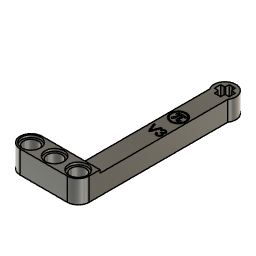
1. Stepper motor holder (L) [V3] (Autodesk Fusion 360 design; units mm, degrees)
Autodesk Fusion 360 part; units mm, degrees
note: some values were not read from the file. Set by a fixed rule: which sketch regions a step uses.
sketch "Base" plane through (0, 0, 0) normal (0, 0, 1) x (1, 0, 0)
  line L0 (3.7, 0) -> (19.7, 0)
  line L1 (19.7, 7.4) -> (3.7, 7.4)
  arc A0 (3.7, 7.4) -> (0, 3.7) centre (3.7, 3.7) ccw
  arc A1 (0, 3.7) -> (3.7, 0) centre (3.7, 3.7) ccw
  arc A2 (19.7, 0) -> (23.4, 3.7) centre (19.7, 3.7) ccw
  circle A3 centre (3.7, 3.7) radius 2.5
  circle A4 centre (3.7, 3.7) radius 3.2
  circle A5 centre (11.7, 3.7) radius 2.5
  circle A6 centre (11.7, 3.7) radius 3.2
  circle A7 centre (19.7, 3.7) radius 2.5
  circle A8 centre (19.7, 3.7) radius 3.2
  line L2 (19.7, 7.4) -> (23.4, 7.4)
  line L3 (23.4, 7.4) -> (23.4, 3.7)
  line L4 (17.85, 52.8) -> (22.85, 52.8)
  line L5 (20.35, 55.3003) -> (20.35, 50.2997)
  line L6 (17.85, 52.8) -> (17.85, 51.75)
  line L7 (19.3, 50.2997) -> (20.35, 50.2997)
  line L8 (20.35, 54.8003) -> (20.35, 0.0575)
  circle A9 centre (20.35, 52.8) radius 3.7125
  line L9 (23.4, 51.75) -> (23.4, 7.4)
  line L10 (17.3, 51.75) -> (17.3, 7.4)
  line L11 (17.85, 51.75) -> (19.05, 51.75)
  line L12 (19.3, 51.5) -> (19.3, 50.2997)
  arc A10 (19.3, 51.5) -> (19.05, 51.75) centre (19.05, 51.5) ccw
  line L13 (22.85, 52.8) -> (22.85, 51.75)
  line L14 (22.85, 51.75) -> (21.65, 51.75)
  arc A11 (21.65, 51.75) -> (21.4, 51.5) centre (21.65, 51.5) ccw
  line L15 (21.4, 51.5) -> (21.4, 50.2997)
  line L16 (21.4, 50.2997) -> (20.35, 50.2997)
  line L17 (17.85, 52.8) -> (17.85, 53.85)
  line L18 (17.85, 53.85) -> (19.05, 53.85)
  arc A12 (19.05, 53.85) -> (19.3, 54.1) centre (19.05, 54.1) ccw
  line L19 (19.3, 54.1) -> (19.3, 55.3003)
  line L20 (19.3, 55.3003) -> (20.35, 55.3003)
  line L21 (21.4, 55.3003) -> (20.35, 55.3003)
  line L22 (21.4, 54.1) -> (21.4, 55.3003)
  arc A13 (21.4, 54.1) -> (21.65, 53.85) centre (21.65, 54.1) ccw
  line L23 (22.85, 53.85) -> (21.65, 53.85)
  line L24 (22.85, 52.8) -> (22.85, 53.85)
  line L25 (17.3, 51.75) -> (17.3, 52.75)
  line L26 (23.4, 51.75) -> (23.4, 52.75)
  arc A14 (20.35, 55.8) -> (17.3, 52.75) centre (20.35, 52.75) ccw
  arc A15 (23.4, 52.75) -> (20.35, 55.8) centre (20.35, 52.75) ccw
  point P0 (23.4, 0)
  point P1 (0, 7.4)
  point P2 (17.3, 54.8)
  point P3 (17.3, 55.8)
  point P4 (23.4, 55.8)
  dimension "d1" = 23.4
  dimension "d2" = 7.4
  dimension "d3" = 3.7
  dimension "d4" = 3.7
  dimension "d6" = 3.7
  dimension "d7" = 5
  dimension "d8" = 6.4
  dimension "d11" = 16
  dimension "d12" = 0
  dimension "d50" = 1.05
  dimension "d51" = 1.05
  dimension "d58" = 0.25
  dimension "d61" = 3.05
  dimension "d62" = 3.05
  constraint horizontal L0
  constraint horizontal L1
  constraint coincident P1 L1
  constraint tangent L1 A0
  constraint coincident origin L0
  constraint tangent L0 A1
  constraint coincident A0.end A1.start
  constraint coincident P0 L0
  constraint tangent L0 A2
  constraint concentric A1 A3
  constraint concentric A0 A4
  constraint horizontal L2
  constraint vertical L3
  constraint midpoint L4 L5
  constraint perpendicular L4 L6
  constraint coincident A2 L8.end
  constraint perpendicular L0 L8
  constraint perpendicular L4 L5
  constraint parallel L5 L8
  constraint midpoint L4 A9.centre
  constraint coincident L1 L10.end
  constraint perpendicular L1 L10
  constraint perpendicular L6 L11
  constraint tangent L11 A10
  constraint tangent L12 A10
  constraint symmetric L4.start L8 L4.end
  constraint symmetric L5.end L8 L7.end
  constraint symmetric L6.end L8 L13.end
  constraint symmetric L7.start L8 L15.end
  constraint symmetric L8 L11.end L14.end
  constraint symmetric L8 L12.start A11.end
  constraint symmetric L8 A10 A11
  constraint symmetric L6.start L4 L17.start
  constraint symmetric L4 L5.end L5.start
  constraint symmetric L4 L6.end L17.end
  constraint symmetric L4 L7.start L19.end
  constraint symmetric L4 L11.end L18.end
  constraint symmetric L4 L12.start A12.end
  constraint symmetric L4 A10 A12
  constraint symmetric L4 L13.start L24.start
  constraint symmetric L4 L13.end L23.start
  constraint symmetric L4 L14.end A13.end
  constraint symmetric L4 A11.end L22.start
  constraint symmetric L4 A11 A13
  constraint symmetric L4 L15.end L21.start
  constraint parallel L10 L25
  constraint parallel L9 L26
  constraint coincident P3 L25
  constraint tangent L25 A14
  constraint coincident P4 L26
  constraint tangent L26 A15
  constraint coincident A14.start A15.end
  measures "d1" distance of origin P0
  measures "d2" distance of origin P1
  measures "d3" radius of A0
  measures "d4" radius of A1
  measures "d6" radius of A2
  measures "d7" diameter of A3
  measures "d8" diameter of A4
  measures "d50" distance of L5.end L7.start
  measures "d51" distance of L4.start L6.end
  measures "d58" radius of A10
  measures "d61" radius of A14
  measures "d62" radius of A15
extrude "Extrude1" add sketch "Base" along normal blind 7.7 contours L0 L1 A0 A1 A2 A8 L2 L8 | A2 A8 L2 L3 L8
extrude "Extrude2" add sketch "Base" along normal blind 6.9 contours A7 A8 L8 | A7 A8 L8 | A4 | A6
extrude "Extrude3" cut sketch "Base" along normal blind 0.8 contours A7 A8 L8 | A7 A8 L8 | A4 | A6
extrude "Extrude4" add sketch "Base" along normal blind 6.7 contours L1 L2 L8 A9 L10 | L2 L8 A9 L9 | A9 L9 L10 L25 L26 A14 A15 | A9 L9 L10 L25 L26 A14 A15
ref_plane "WorkPlane1" through (20.35, 32.5818, 6.7) normal (0, 0, 1) x (1, 0, 0)
sketch "Author" plane through (0, 0, 6.7) normal (0, 0, 1) x (1, 0, 0)
  line L0 (18.8552, 37.6405) -> (18.9613, 37.6326)
  spline S0 degree 3 poles (18.9613, 37.6326) (19.0712, 37.757) (19.1144, 38.1249) (19.7625, 38.0529) knots 0 0 0 0 1 1 1 1
  spline S1 degree 3 poles (19.7625, 38.0529) (19.7389, 36.4766) (19.0477, 36.3103) (19.0909, 35.9869) knots 0 0 0 0 1 1 1 1
  spline S2 degree 3 poles (19.0909, 35.9869) (19.1066, 35.8036) (19.2519, 35.691) (19.409, 35.6845) knots 0 0 0 0 1 1 1 1
  spline S3 degree 3 poles (19.409, 35.6845) (19.9052, 35.7015) (19.883, 36.3705) (20.0374, 38.0568) knots 0 0 0 0 1 1 1 1
  line L1 (20.0374, 38.0568) -> (20.6777, 38.0568)
  spline S4 degree 3 poles (20.6777, 38.0568) (20.6436, 37.4624) (20.5507, 36.868) (20.5402, 36.2854) knots 0 0 0 0 1 1 1 1
  spline S5 degree 3 poles (20.5402, 36.2854) (20.548, 35.8979) (20.7837, 35.691) (21.094, 35.6884) knots 0 0 0 0 1 1 1 1
  spline S6 degree 3 poles (21.094, 35.6884) (21.6046, 35.6714) (21.7656, 36.2671) (21.7656, 36.5211) knots 0 0 0 0 1 1 1 1
  line L2 (21.7656, 36.5211) -> (21.6556, 36.5211)
  spline S7 degree 3 poles (21.6556, 36.5211) (21.6452, 36.3116) (21.5444, 36.161) (21.3297, 36.1519) knots 0 0 0 0 1 1 1 1
  spline S8 degree 3 poles (21.3297, 36.1519) (20.7444, 36.144) (21.0665, 37.1809) (21.0704, 38.0489) knots 0 0 0 0 1 1 1 1
  line L3 (21.0704, 38.0489) -> (21.7656, 38.045)
  line L4 (21.7656, 38.045) -> (21.7617, 38.4888)
  spline S9 degree 3 poles (21.7617, 38.4888) (18.8722, 38.5028) (19.2389, 38.5595) (18.8552, 37.6405) knots 0 0 0 0 1 1 1 1
  arc A0 (17.6646, 37.0896) -> (20.3104, 39.7354) centre (20.3104, 37.0896) cw
  arc A1 (20.3104, 34.4438) -> (17.6646, 37.0896) centre (20.3104, 37.0896) cw
  arc A2 (22.9562, 37.0896) -> (20.3104, 34.4438) centre (20.3104, 37.0896) cw
  arc A3 (20.3104, 39.7354) -> (22.9562, 37.0896) centre (20.3104, 37.0896) cw
  arc A4 (20.3104, 39.3815) -> (20.3694, 39.3807) centre (20.3107, 37.0896) cw
  arc A5 (20.3694, 39.3807) -> (20.4284, 39.3784) centre (20.3103, 37.0896) cw
  arc A6 (20.4284, 39.3784) -> (20.4873, 39.3746) centre (20.3102, 37.0896) cw
  arc A7 (20.4873, 39.3746) -> (20.5461, 39.3693) centre (20.3107, 37.0896) cw
  arc A8 (20.5461, 39.3693) -> (20.6047, 39.3625) centre (20.3104, 37.0896) cw
  arc A9 (20.6047, 39.3625) -> (20.6631, 39.3542) centre (20.3106, 37.0896) cw
  arc A10 (20.6631, 39.3542) -> (20.7213, 39.3443) centre (20.3099, 37.0897) cw
  arc A11 (20.7213, 39.3443) -> (20.7792, 39.333) centre (20.3106, 37.0895) cw
  arc A12 (20.7792, 39.333) -> (20.8368, 39.3202) centre (20.3106, 37.0895) cw
  arc A13 (20.8368, 39.3202) -> (20.8941, 39.3059) centre (20.31, 37.0897) cw
  arc A14 (20.8941, 39.3059) -> (20.951, 39.2901) centre (20.3109, 37.0894) cw
  arc A15 (20.951, 39.2901) -> (21.0074, 39.2729) centre (20.3102, 37.0897) cw
  arc A16 (21.0074, 39.2729) -> (21.0634, 39.2542) centre (20.3102, 37.0896) cw
  arc A17 (21.0634, 39.2542) -> (21.1189, 39.2341) centre (20.3106, 37.0895) cw
  arc A18 (21.1189, 39.2341) -> (21.1738, 39.2126) centre (20.3102, 37.0897) cw
  arc A19 (21.1738, 39.2126) -> (21.2282, 39.1897) centre (20.3106, 37.0895) cw
  arc A20 (21.2282, 39.1897) -> (21.282, 39.1653) centre (20.3106, 37.0895) cw
  arc A21 (21.282, 39.1653) -> (21.3351, 39.1396) centre (20.3103, 37.0896) cw
  arc A22 (21.3351, 39.1396) -> (21.3875, 39.1126) centre (20.3106, 37.0895) cw
  arc A23 (21.3875, 39.1126) -> (21.4393, 39.0842) centre (20.3101, 37.0898) cw
  arc A24 (21.4393, 39.0842) -> (21.4903, 39.0544) centre (20.3105, 37.0895) cw
  arc A25 (21.4903, 39.0544) -> (21.5405, 39.0234) centre (20.3103, 37.0896) cw
  arc A26 (21.5405, 39.0234) -> (21.5898, 38.9911) centre (20.3103, 37.0897) cw
  arc A27 (21.5898, 38.9911) -> (21.6384, 38.9575) centre (20.3106, 37.0894) cw
  arc A28 (21.6384, 38.9575) -> (21.686, 38.9227) centre (20.3106, 37.0895) cw
  arc A29 (21.686, 38.9227) -> (21.7328, 38.8867) centre (20.3102, 37.0897) cw
  arc A30 (21.7328, 38.8867) -> (21.7786, 38.8495) centre (20.3105, 37.0895) cw
  arc A31 (21.7786, 38.8495) -> (21.8234, 38.8111) centre (20.3104, 37.0896) cw
  arc A32 (21.8234, 38.8111) -> (21.8672, 38.7716) centre (20.3104, 37.0896) cw
  arc A33 (21.8672, 38.7716) -> (21.91, 38.7309) centre (20.3106, 37.0894) cw
  arc A34 (21.91, 38.7309) -> (21.9518, 38.6892) centre (20.3104, 37.0896) cw
  arc A35 (21.9518, 38.6892) -> (21.9924, 38.6464) centre (20.3102, 37.0898) cw
  arc A36 (21.9924, 38.6464) -> (22.0319, 38.6026) centre (20.3105, 37.0895) cw
  arc A37 (22.0319, 38.6026) -> (22.0703, 38.5577) centre (20.3105, 37.0895) cw
  arc A38 (22.0703, 38.5577) -> (22.1075, 38.5119) centre (20.3103, 37.0897) cw
  arc A39 (22.1075, 38.5119) -> (22.1436, 38.4652) centre (20.3106, 37.0894) cw
  arc A40 (22.1436, 38.4652) -> (22.1784, 38.4175) centre (20.3103, 37.0897) cw
  arc A41 (22.1784, 38.4175) -> (22.2119, 38.369) centre (20.3103, 37.0898) cw
  arc A42 (22.2119, 38.369) -> (22.2442, 38.3196) centre (20.3105, 37.0895) cw
  arc A43 (22.2442, 38.3196) -> (22.2753, 38.2694) centre (20.3105, 37.0895) cw
  arc A44 (22.2753, 38.2694) -> (22.305, 38.2184) centre (20.3103, 37.0897) cw
  arc A45 (22.305, 38.2184) -> (22.3334, 38.1667) centre (20.3106, 37.0892) cw
  arc A46 (22.3334, 38.1667) -> (22.3605, 38.1143) centre (20.3103, 37.0898) cw
  arc A47 (22.3605, 38.1143) -> (22.3862, 38.0611) centre (20.3105, 37.0895) cw
  arc A48 (22.3862, 38.0611) -> (22.4105, 38.0074) centre (20.3103, 37.0898) cw
  arc A49 (22.4105, 38.0074) -> (22.4334, 37.953) centre (20.3105, 37.0893) cw
  arc A50 (22.4334, 37.953) -> (22.455, 37.898) centre (20.3103, 37.0898) cw
  arc A51 (22.455, 37.898) -> (22.4751, 37.8426) centre (20.3103, 37.0898) cw
  arc A52 (22.4751, 37.8426) -> (22.4937, 37.7866) centre (20.3105, 37.0894) cw
  arc A53 (22.4937, 37.7866) -> (22.511, 37.7301) centre (20.3105, 37.0893) cw
  arc A54 (22.511, 37.7301) -> (22.5267, 37.6733) centre (20.3103, 37.0901) cw
  arc A55 (22.5267, 37.6733) -> (22.541, 37.616) centre (20.3105, 37.0892) cw
  arc A56 (22.541, 37.616) -> (22.5538, 37.5584) centre (20.3104, 37.0898) cw
  arc A57 (22.5538, 37.5584) -> (22.5652, 37.5005) centre (20.3105, 37.0893) cw
  arc A58 (22.5652, 37.5005) -> (22.575, 37.4423) centre (20.3104, 37.0896) cw
  arc A59 (22.575, 37.4423) -> (22.5833, 37.3839) centre (20.3104, 37.0897) cw
  arc A60 (22.5833, 37.3839) -> (22.5901, 37.3252) centre (20.3104, 37.0896) cw
  arc A61 (22.5901, 37.3252) -> (22.5954, 37.2665) centre (20.3104, 37.0899) cw
  arc A62 (22.5954, 37.2665) -> (22.5993, 37.2076) centre (20.3104, 37.0894) cw
  arc A63 (22.5993, 37.2076) -> (22.6015, 37.1486) centre (20.3104, 37.0894) cw
  arc A64 (22.6015, 37.1486) -> (22.6023, 37.0896) centre (20.3104, 37.0899) cw
  arc A65 (22.6023, 37.0896) -> (22.5959, 36.9183) centre (20.3104, 37.0895) cw
  arc A66 (22.5959, 36.9183) -> (22.5767, 36.748) centre (20.3104, 37.0897) cw
  arc A67 (22.5767, 36.748) -> (22.5448, 36.5796) centre (20.3104, 37.0895) cw
  arc A68 (22.5448, 36.5796) -> (22.5005, 36.414) centre (20.3104, 37.0897) cw
  arc A69 (22.5005, 36.414) -> (22.4439, 36.2523) centre (20.3104, 37.0896) cw
  arc A70 (22.4439, 36.2523) -> (22.3753, 36.0952) centre (20.3104, 37.0896) cw
  arc A71 (22.3753, 36.0952) -> (22.2952, 35.9436) centre (20.3104, 37.0895) cw
  arc A72 (22.2952, 35.9436) -> (22.2041, 35.7985) centre (20.3104, 37.0896) cw
  arc A73 (22.2041, 35.7985) -> (22.1023, 35.6606) centre (20.3104, 37.0896) cw
  arc A74 (22.1023, 35.6606) -> (21.9905, 35.5307) centre (20.3104, 37.0896) cw
  arc A75 (21.9905, 35.5307) -> (21.8693, 35.4095) centre (20.3103, 37.0895) cw
  arc A76 (21.8693, 35.4095) -> (21.7394, 35.2977) centre (20.3105, 37.0897) cw
  arc A77 (21.7394, 35.2977) -> (21.6015, 35.1959) centre (20.3104, 37.0896) cw
  arc A78 (21.6015, 35.1959) -> (21.4563, 35.1048) centre (20.3104, 37.0896) cw
  arc A79 (21.4563, 35.1048) -> (21.3048, 35.0247) centre (20.3104, 37.0896) cw
  arc A80 (21.3048, 35.0247) -> (21.1477, 34.9561) centre (20.3104, 37.0896) cw
  arc A81 (21.1477, 34.9561) -> (20.986, 34.8995) centre (20.3104, 37.0896) cw
  arc A82 (20.986, 34.8995) -> (20.8204, 34.8552) centre (20.3103, 37.0896) cw
  arc A83 (20.8204, 34.8552) -> (20.652, 34.8233) centre (20.3105, 37.0896) cw
  arc A84 (20.652, 34.8233) -> (20.4817, 34.8041) centre (20.3103, 37.0896) cw
  arc A85 (20.4817, 34.8041) -> (20.3104, 34.7977) centre (20.3105, 37.0896) cw
  arc A86 (20.3104, 34.7977) -> (20.1391, 34.8041) centre (20.3103, 37.0896) cw
  arc A87 (20.1391, 34.8041) -> (19.9688, 34.8233) centre (20.3105, 37.0896) cw
  arc A88 (19.9688, 34.8233) -> (19.8004, 34.8552) centre (20.3104, 37.0896) cw
  arc A89 (19.8004, 34.8552) -> (19.6349, 34.8995) centre (20.3105, 37.0896) cw
  arc A90 (19.6349, 34.8995) -> (19.4731, 34.9561) centre (20.3104, 37.0896) cw
  arc A91 (19.4731, 34.9561) -> (19.316, 35.0247) centre (20.3104, 37.0896) cw
  arc A92 (19.316, 35.0247) -> (19.1645, 35.1048) centre (20.3104, 37.0896) cw
  arc A93 (19.1645, 35.1048) -> (19.0194, 35.1959) centre (20.3104, 37.0896) cw
  arc A94 (19.0194, 35.1959) -> (18.8815, 35.2977) centre (20.3104, 37.0896) cw
  arc A95 (18.8815, 35.2977) -> (18.7515, 35.4095) centre (20.3103, 37.0897) cw
  arc A96 (18.7515, 35.4095) -> (18.6303, 35.5307) centre (20.3104, 37.0896) cw
  arc A97 (18.6303, 35.5307) -> (18.5186, 35.6606) centre (20.3105, 37.0895) cw
  arc A98 (18.5186, 35.6606) -> (18.4168, 35.7985) centre (20.3104, 37.0896) cw
  arc A99 (18.4168, 35.7985) -> (18.3256, 35.9436) centre (20.3104, 37.0896) cw
  arc A100 (18.3256, 35.9436) -> (18.2455, 36.0952) centre (20.3105, 37.0895) cw
  arc A101 (18.2455, 36.0952) -> (18.177, 36.2523) centre (20.3104, 37.0896) cw
  arc A102 (18.177, 36.2523) -> (18.1204, 36.414) centre (20.3104, 37.0896) cw
  arc A103 (18.1204, 36.414) -> (18.076, 36.5796) centre (20.3104, 37.0897) cw
  arc A104 (18.076, 36.5796) -> (18.0441, 36.748) centre (20.3104, 37.0895) cw
  arc A105 (18.0441, 36.748) -> (18.0249, 36.9183) centre (20.3104, 37.0897) cw
  arc A106 (18.0249, 36.9183) -> (18.0185, 37.0896) centre (20.3104, 37.0895) cw
  arc A107 (18.0185, 37.0896) -> (18.0249, 37.2609) centre (20.3104, 37.0897) cw
  arc A108 (18.0249, 37.2609) -> (18.0441, 37.4312) centre (20.3104, 37.0895) cw
  arc A109 (18.0441, 37.4312) -> (18.076, 37.5996) centre (20.3104, 37.0897) cw
  arc A110 (18.076, 37.5996) -> (18.1204, 37.7651) centre (20.3104, 37.0895) cw
  arc A111 (18.1204, 37.7651) -> (18.177, 37.9269) centre (20.3104, 37.0896) cw
  arc A112 (18.177, 37.9269) -> (18.2455, 38.084) centre (20.3104, 37.0896) cw
  arc A113 (18.2455, 38.084) -> (18.3256, 38.2355) centre (20.3104, 37.0896) cw
  arc A114 (18.3256, 38.2355) -> (18.4168, 38.3806) centre (20.3104, 37.0896) cw
  arc A115 (18.4168, 38.3806) -> (18.5186, 38.5185) centre (20.3104, 37.0896) cw
  arc A116 (18.5186, 38.5185) -> (18.6303, 38.6485) centre (20.3105, 37.0897) cw
  arc A117 (18.6303, 38.6485) -> (18.7515, 38.7696) centre (20.3103, 37.0895) cw
  arc A118 (18.7515, 38.7696) -> (18.8815, 38.8814) centre (20.3104, 37.0896) cw
  arc A119 (18.8815, 38.8814) -> (19.0194, 38.9832) centre (20.3104, 37.0896) cw
  arc A120 (19.0194, 38.9832) -> (19.1645, 39.0744) centre (20.3104, 37.0896) cw
  arc A121 (19.1645, 39.0744) -> (19.316, 39.1545) centre (20.3104, 37.0896) cw
  arc A122 (19.316, 39.1545) -> (19.4731, 39.223) centre (20.3104, 37.0896) cw
  arc A123 (19.4731, 39.223) -> (19.6349, 39.2796) centre (20.3104, 37.0896) cw
  arc A124 (19.6349, 39.2796) -> (19.8004, 39.324) centre (20.3105, 37.0896) cw
  arc A125 (19.8004, 39.324) -> (19.9688, 39.3559) centre (20.3104, 37.0896) cw
  arc A126 (19.9688, 39.3559) -> (20.1391, 39.3751) centre (20.3105, 37.0896) cw
  arc A127 (20.1391, 39.3751) -> (20.3104, 39.3815) centre (20.3103, 37.0896) cw
extrude "Extrude5" cut sketch "Author" against normal blind 0.6
sketch "Version" plane through (0, 0, 6.7) normal (0, 0, 1) x (-1, 0, 0)
  line L0 (-17.3, -7.4) -> (-23.4, -7.4)
  arc A0 (-20.3104, -34.4438) -> (-22.9562, -37.0896) centre (-20.3104, -37.0896) ccw
  arc A1 (-22.9563, -37.0896) -> (-20.3104, -34.4437) centre (-20.3104, -37.0896) ccw
  line L1 (-18, -28.0896) -> (-23, -28.0896) construction
  line L2 (-23, -28.0896) -> (-23, -31.0896) construction
  line L3 (-23, -31.0896) -> (-18, -31.0896) construction
  line L4 (-18, -31.0896) -> (-18, -28.0896) construction
  arc A2 (-23.4, -49.6834) -> (-17.3, -49.6834) centre (-20.35, -51.8) ccw
  line L5 (-17.3, -49.6834) -> (-17.3, -7.4)
  line L6 (-23.4, -7.4) -> (-23.4, -49.6834)
  line L7 (-22.85, -52.85) -> (-22.85, -50.75)
  line L8 (-22.85, -50.75) -> (-21.7, -50.75)
  arc A3 (-21.7, -50.75) -> (-21.4, -50.45) centre (-21.7, -50.45) ccw
  line L9 (-21.4, -50.45) -> (-21.4, -49.2997)
  line L10 (-21.4, -49.2997) -> (-20.35, -49.2997)
  line L11 (-20.35, -49.2997) -> (-19.3, -49.2997)
  line L12 (-19.3, -49.2997) -> (-19.3, -50.45)
  arc A4 (-19.3, -50.45) -> (-19, -50.75) centre (-19, -50.45) ccw
  line L13 (-19, -50.75) -> (-17.85, -50.75)
  line L14 (-17.85, -50.75) -> (-17.85, -52.85)
  line L15 (-17.85, -52.85) -> (-19, -52.85)
  arc A5 (-19, -52.85) -> (-19.3, -53.15) centre (-19, -53.15) ccw
  line L16 (-19.3, -53.15) -> (-19.3, -54.3003)
  line L17 (-19.3, -54.3003) -> (-20.35, -54.3003)
  line L18 (-20.35, -54.3003) -> (-21.4, -54.3003)
  line L19 (-21.4, -54.3003) -> (-21.4, -53.15)
  arc A6 (-21.4, -53.15) -> (-21.7, -52.85) centre (-21.7, -53.15) ccw
  line L20 (-21.7, -52.85) -> (-22.85, -52.85)
  line L21 (-20.5, -31.0896) -> (-20.5, -28.0896)
  line L22 (-18, -29.5896) -> (-23, -29.5896)
  point P0 (-20.3103, -37.0896)
  point P1 (-20.35, -51.75)
  dimension "d38" = 3
  dimension "d55" = 14.6604
  dimension "d56" = 6
  text T0 "V3" font "Arial" height 3 align left top in box 5 x 3 at (-18, -28.0896) x (-1, 0) y (0, -1) spacing 1
  constraint coincident L21.start
  constraint midpoint L1 L21.end
  constraint perpendicular L1 L21
  constraint midpoint L4 L22.start
  constraint midpoint L2 L22.end
  measures "d55" vertical distance of P0 P1
  measures "d56" vertical distance of P0 L21.start
extrude "Extrude6" cut sketch "Version" against normal blind 0.6 text T0
named bodies: "Base"
